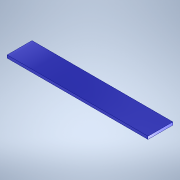
# Autodesk Inventor part: Antenna
Saved by Autodesk Inventor 2020 (Build 240168000, 168)
## iProperties
Created: 2021-10-31
Part Number: Antenna
Material: 一般
Document SubType Name: Modeling
Designer: Masato Kubotera
Density: 1 g/cm^3
Appearance: 青 - 壁塗料 - 光沢
Description: 既製品
Author: Masato Kubotera
Autodesk Inventor part; units mm, degrees
ref_plane "YZ Plane" through (0, 0, 0) normal (1, 0, 0) x (0, 1, 0)
ref_plane "XZ Plane" through (0, 0, 0) normal (0, 1, 0) x (-1, 0, 0)
ref_plane "XY Plane" through (0, 0, 0) normal (0, 0, 1) x (1, 0, 0)
sketch "スケッチ1" plane through (0, 0, 0) normal (0, 0, 1) x (1, 0, 0)
  line L0 (-25.5, 4.5) -> (25.5, 4.5)
  line L1 (25.5, 4.5) -> (25.5, -4.5)
  line L2 (25.5, -4.5) -> (-25.5, -4.5)
  line L3 (-25.5, -4.5) -> (-25.5, 4.5)
  line L4 (-25.5, 4.5) -> (25.5, -4.5) construction
  line L5 (25.5, 4.5) -> (-25.5, -4.5) construction
  point P0 (0, 0)
  dimension "d0" = 51
  dimension "d1" = 9
  constraints: 12 end point, 2 midpoint, 2 parallel, 1 horizontal, 1 perpendicular
  measures "d0" distance of L1.end L2.end
  measures "d1" distance of L0.end L1.end
extrude "押し出し1" add sketch "スケッチ1" along normal blind 1
